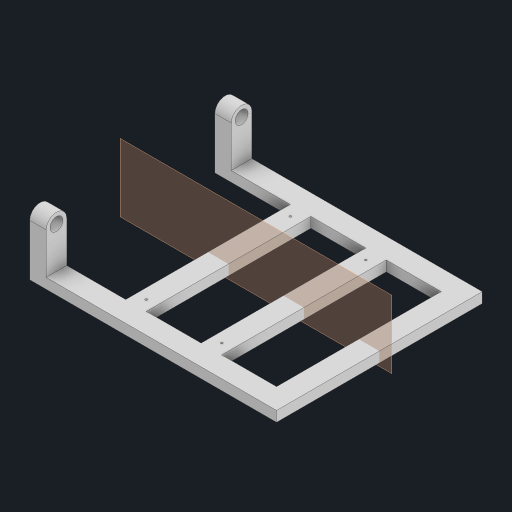
# Autodesk Inventor part: table_base
Saved by Autodesk Inventor 2024 (Build 280153000, 153)
## iProperties
Created: 2024-06-21
Part Number: table_base
Material: Generic
Document SubType Name: Modeling
Designer: mihir
Density: 1 g/cm^3
Appearance: Default
Author: mihir
Autodesk Inventor part; units mm, degrees
ref_plane "YZ Plane" through (0, 0, 0) normal (1, 0, 0) x (0, 1, 0)
ref_plane "XZ Plane" through (0, 0, 0) normal (0, 1, 0) x (-1, 0, 0)
ref_plane "XY Plane" through (0, 0, 0) normal (0, 0, 1) x (1, 0, 0)
sketch "Sketch1" plane through (0, 0, 0) normal (0, 1, 0) x (-1, 0, 0)
  line L0 (0, 0) -> (0, -100)
  line L1 (0, -100) -> (120, -100)
  line L2 (120, -100) -> (120, -90)
  line L3 (120, -90) -> (83.3333, -90)
  line L4 (83.3333, -90) -> (83.3333, -10)
  line L5 (83.3333, -10) -> (120, -10)
  line L6 (120, -10) -> (120, 0)
  line L7 (120, 0) -> (0, 0)
  line L8 (73.3333, -10) -> (46.6667, -10)
  line L9 (46.6667, -10) -> (46.6667, -90)
  line L10 (46.6667, -90) -> (73.3333, -90)
  line L11 (73.3333, -90) -> (73.3333, -10)
  line L12 (36.6667, -10) -> (10, -10)
  line L13 (10, -10) -> (10, -90)
  line L14 (10, -90) -> (36.6667, -90)
  line L15 (36.6667, -90) -> (36.6667, -10)
  dimension "d1" = 120
  dimension "d2" = 10
  dimension "d3" = 100
  dimension "d4" = 10
  dimension "d5" = 10
  dimension "d6" = 10
  dimension "d16" = 26.6667
  constraints: 32 end point, 8 perpendicular, 4 parallel, 4 point on line, 3 equal length, 2 horizontal, 1 collinear, 1 vertical
  measures "d1" distance of L0.end L1.end
  measures "d2" distance of L5.end L6.end
  measures "d3" distance of L0.start L0.end
  measures "d4" distance between parallel lines of L4 L11
  measures "d5" distance between parallel lines of L0 L13
  measures "d6" distance between parallel lines of L9 L15
  measures "d16" distance of L13.end L14.end
extrude "Extrusion1" add sketch "Sketch1" along normal blind 5
sketch "Sketch2" plane through (-120, 0, -10) normal (-1, 0, 0) x (0, 0, 1)
  line L0 (0, 0) -> (0, 5) projected
  line L1 (0, 0) -> (10, 0)
  line L2 (10, 0) -> (10, 25)
  line L3 (10, 25) -> (0, 25)
  line L4 (0, 25) -> (0, 0)
  circle A0 centre (5, 25) radius 3.15
  arc A1 (10, 25) -> (0, 25) centre (5, 25) ccw
  line L5 (10, 0) -> (10, 5) projected
  point P0 (0, 5)
  dimension "d9" = 25
  dimension "d10" = 6.3
  constraints: 8 end point, 2 centre point, 2 parallel, 2 point on circle, 1 coincident, 1 collinear, 1 horizontal, 1 midpoint, 1 perpendicular
  measures "d9" distance of L1.end L2.end
  measures "d10" diameter of A0
extrude "Extrusion2" add sketch "Sketch2" against normal blind 8
sketch "Sketch3" plane through (-112, 0, -10) normal (1, 0, 0) x (0, 0, -1)
  arc A0 (0, 25) -> (-10, 25) centre (-5, 25) ccw projected
  circle A1 centre (-5, 25) radius 3.15
  point P0 (-10, 0)
  dimension "d13" = 6.3
  constraints: 1 centre point, 1 coincident
  measures "d13" diameter of A1
extrude "Extrusion3" cut sketch "Sketch3" against normal blind 6
ref_plane "Work Plane1" through (-120, 0, -50) normal (0, 0, 1) x (1, 0, 0)
mirror "Mirror1" about plane through (-120, 0, -50) normal (0, 0, 1) of "Extrusion2", "Extrusion3"
sketch "Sketch4" plane through (0, 5, 0) normal (0, 1, 0) x (1, 0, 0)
  line L0 (-83.3333, 90) -> (-83.3333, 10) projected
  line L1 (-112, 0) -> (0, 0) projected
  point P0 (-78.3333, 15)
  point P1 (-41.6667, 15)
  point P2 (-78.3333, 85)
  point P3 (-41.6667, 85)
  dimension "d17" = 5
  dimension "d18" = 15
  dimension "d21" = 36.6667
  dimension "d24" = 70
  constraints: 1 horizontal, 1 vertical, 3 other
  measures "d17" distance from line of L0 point (-78.333, 15)
  measures "d18" distance from line of L1 point (-78.333, 15)
  measures "d21" distance of point (-78.333, 15) point (-41.667, 15)
  measures "d24" distance of point (-78.333, 15) point (-78.333, 85)
hole "Hole1" at (-78.3333, 5, -15) at (-41.6667, 5, -15) at (-78.3333, 5, -85) at (-41.6667, 5, -85) direction (0, -1, 0) diameter 1 end through all
equation "\"d1\" = table_base_length"
equation "\"d2\" = table_base_web_width"
equation "\"d3\" = table_base_width"
equation "\"d4\" = table_base_web_width"
equation "\"d5\" = table_base_web_width"
equation "\"d6\" = table_base_web_width"
equation "\"d16\" = -1.33333 * table_base_web_width + 0.333333 * table_base_length"
equation "\"d7\" = table_base_thickness"
equation "\"d9\" = table_base_rod_height"
equation "\"d10\" = rod_diameter + rod_tolerance"
equation "\"d11\" = table_base_rod_holder_thickness"
equation "\"d13\" = rod_diameter + rod_tolerance"
equation "\"d14\" = 0.75 * table_base_rod_holder_thickness"
equation "\"d17\" = 0.5 * table_base_web_width"
equation "\"d18\" = 1.5 * table_base_web_width"
equation "\"d21\" = -0.333333 * table_base_web_width + 0.333333 * table_base_length"
equation "\"d24\" = table_base_width - 3 * table_base_web_width"
equation "\"d27\" = screw_diameter"
equation "\"table_base_length\" = 120"
equation "\"table_base_width\" = 100"
equation "\"table_base_thickness\" = 5"
equation "\"table_base_web_width\" = 10"
equation "\"table_base_rod_height\" = 25"
equation "\"rod_diameter\" = 6"
equation "\"rod_tolerance\" = 0.3"
equation "\"table_base_rod_holder_thickness\" = 8"
equation "\"screw_diameter\" = 1"
body "Solid1"
